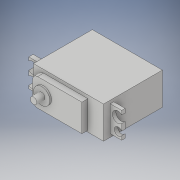
# Autodesk Inventor part: sorting
Saved by Autodesk Inventor 2019 (Build 230136000, 136)
## iProperties
Created: 2020-02-29
Part Number: sorting
Material: Generic
Document SubType Name: Modeling
Designer: VIGNESH
Density: 1 g/cm^3
Appearance: Default
Author: VIGNESH
Autodesk Inventor part; units mm, degrees
ref_plane "YZ Plane" through (0, 0, 0) normal (1, 0, 0) x (0, 1, 0)
ref_plane "XZ Plane" through (0, 0, 0) normal (0, 1, 0) x (-1, 0, 0)
ref_plane "XY Plane" through (0, 0, 0) normal (0, 0, 1) x (1, 0, 0)
sketch "Sketch1" plane through (0, 0, 0) normal (0, 0, 1) x (1, 0, 0)
  line L0 (0, 0) -> (42.9, 0)
  line L1 (42.9, 0) -> (42.9, 19.7)
  line L2 (42.9, 19.7) -> (0, 19.7)
  line L3 (0, 19.7) -> (0, 0)
  dimension "d0" = 42.9
  dimension "d1" = 19.7
  constraints: 8 end point, 2 parallel, 1 horizontal, 1 perpendicular
  measures "d0" distance of L2.end L1.end
  measures "d1" distance of L1.end L0.end
extrude "Extrusion1" add sketch "Sketch1" along normal blind 36
sketch "Sketch2" plane through (0, 0, 36) normal (0, 0, 1) x (1, 0, 0)
  line L0 (3.1975, 17.7737) -> (33.3653, 17.7737)
  line L1 (33.3653, 17.7737) -> (33.3653, 1.0692)
  line L2 (33.3653, 1.0692) -> (3.1975, 1.0692)
  line L3 (3.1975, 1.0692) -> (3.1975, 17.7737)
  point P0 (0, 0)
  constraints: 8 end point, 2 parallel, 1 horizontal, 1 perpendicular
extrude "Extrusion2" add sketch "Sketch2" along normal blind 3.7
fillet "Fillet1" radius 3 1 edges at (3.1975, 1.0692, 37.85)
fillet "Fillet2" radius 3 1 edges at (3.1975, 17.7737, 37.85)
sketch "Sketch3" plane through (0, 0, 39.7) normal (0, 0, 1) x (1, 0, 0)
  circle A0 centre (9.7525, 9.7525) radius 5
  point P0 (0, 0)
  dimension "d8" = 10
  constraints: 1 centre point
  measures "d8" diameter of A0
extrude "Extrusion3" add sketch "Sketch3" along normal blind 1
sketch "Sketch4" plane through (9.7525, 9.7525, 40.7) normal (0, 0, 1) x (1, 0, 0)
  circle A0 centre (0, 0) radius 2
  point P0 (-9.7525, -9.7525)
  dimension "d11" = 4
  constraints: 1 centre point
  measures "d11" diameter of A0
extrude "Extrusion4" add sketch "Sketch4" along normal blind 5
sketch "Sketch5" plane through (0, 0, 0) normal (-1, 0, 0) x (0, 0, 1)
  line L0 (31.9055, 17.6776) -> (29.163, 17.6776)
  line L1 (29.163, 17.6776) -> (29.163, 0.8485)
  line L2 (29.163, 0.8485) -> (31.9055, 0.8485)
  line L3 (31.9055, 0.8485) -> (31.9055, 17.6776)
  point P0 (0, 0)
  constraints: 8 end point, 2 parallel, 1 horizontal, 1 perpendicular
extrude "Extrusion5" add sketch "Sketch5" along normal blind 7
sketch "Sketch6" plane through (0, 0.8485, 31.9055) normal (0, 0, 1) x (1, 0, 0)
  circle A0 centre (-4.7474, 12.2898) radius 3.3866
  point P0 (0, -0.8485)
  constraints: 1 centre point
extrude "Extrusion6" cut sketch "Sketch6" against normal through all
sketch "Sketch7" plane through (0, 0.8485, 31.9055) normal (0, 0, 1) x (1, 0, 0)
  circle A0 centre (-5.0418, 4.3406) radius 3.2151
  point P0 (0, -0.8485)
  constraints: 1 centre point
extrude "Extrusion7" cut sketch "Sketch7" against normal blind 7
sketch "Sketch8" plane through (42.9, 0, 0) normal (1, 0, 0) x (0, 0, -1)
  line L0 (-31.9055, 1.974) -> (-31.9055, 8.4041) projected
  line L1 (-31.9055, 1.974) -> (-29.7764, 1.974)
  line L2 (-29.7764, 1.974) -> (-29.7764, 17.7891)
  line L3 (-29.7764, 17.7891) -> (-31.9055, 17.7891)
  line L4 (-31.9055, 17.7891) -> (-31.9055, 1.974)
  point P0 (0, 0)
  point P1 (-31.9055, 7.739)
  point P2 (-31.9055, 2.6391)
  constraints: 8 end point, 2 parallel, 1 horizontal, 1 perpendicular
extrude "Extrusion8" add sketch "Sketch8" along normal blind 7
sketch "Sketch9" plane through (42.9, 1.974, 31.9055) normal (0, 0, 1) x (1, 0, 0)
  circle A0 centre (4.9018, 3.5919) radius 2.4255
  point P0 (-42.9, -1.974)
  constraints: 1 centre point
extrude "Extrusion9" cut sketch "Sketch9" against normal blind 7
sketch "Sketch10" plane through (42.9, 1.974, 31.9055) normal (0, 0, 1) x (1, 0, 0)
  circle A0 centre (4.6112, 11.0906) radius 3.2917
  point P0 (-42.9, -1.974)
  constraints: 1 centre point
extrude "Extrusion10" cut sketch "Sketch10" against normal blind 7
sketch "Sketch11" plane through (0, 0, 36) normal (0, 0, 1) x (1, 0, 0)
  point P0 (0, 0)
body "Solid1"
